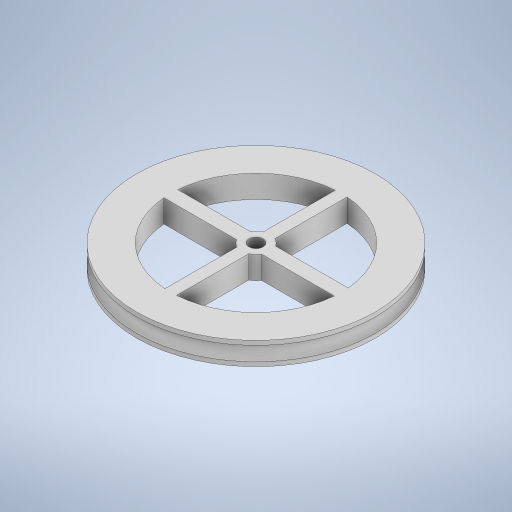
# Autodesk Inventor part: Roue_pami_V3
Saved by Autodesk Inventor 2023 (Build 270158000, 158)
## iProperties
Created: 2024-02-08
Part Number: Roue_pami_V3
Material: Generic
Document SubType Name: Modeling
Designer: eliott
Density: 1 g/cm^3
Appearance: Default
Author: eliott
Autodesk Inventor part; units mm, degrees
ref_plane "YZ Plane" through (0, 0, 0) normal (1, 0, 0) x (0, 1, 0)
ref_plane "XZ Plane" through (0, 0, 0) normal (0, 1, 0) x (-1, 0, 0)
ref_plane "XY Plane" through (0, 0, 0) normal (0, 0, 1) x (1, 0, 0)
sketch "Sketch1" plane through (0, 0, 0) normal (0, 0, 1) x (1, 0, 0)
  line L0 (0, 0) -> (2.5, 0)
  line L1 (2.5, 0) -> (2.5, 8)
  line L2 (2.5, 8) -> (0, 8)
  line L3 (0, 8) -> (0, 0)
  line L4 (2.5, 8) -> (42, 8)
  line L5 (42, 8) -> (42, 0)
  line L6 (42, 0) -> (2.5, 0)
  line L7 (2.5, 0) -> (2.5, 8)
  circle A0 centre (42, 4) radius 2.5
  point P0 (42, 1.5)
  point P1 (42, 6.5)
  dimension "d0" = 8
  dimension "d1" = 2.5
  dimension "d2" = 39.5
  dimension "d3" = 5
  constraints: 16 end point, 4 parallel, 2 horizontal, 2 perpendicular, 1 centre point, 1 midpoint
  measures "d0" distance of L0.end L1.end
  measures "d1" distance of L1.end L2.end
  measures "d2" distance of L1.end L4.end
  measures "d3" diameter of A0
revolve "Revolution1" add sketch "Sketch1" angle 360 about axis through (0, 8, 0) along (0, -1, 0) contours L1 L4 L5 A0 L6
sketch "Sketch2" plane through (0, 8, 0) normal (0, 1, 0) x (1, 0, 0)
  circle A0 centre (0, 0) radius 2.5 projected
  circle A1 centre (0, 0) radius 30
  circle A2 centre (0, 0) radius 5
  line L0 (-4.3623, -2.4434) -> (-29.9003, -2.4434)
  line L1 (-4.3623, 2.4434) -> (-29.9003, 2.4434)
  line L2 (4.3623, 2.4434) -> (29.9003, 2.4434)
  line L3 (4.3623, -2.4434) -> (29.9003, -2.4434)
  line L4 (2.0546, -4.5583) -> (2.0546, -29.9296)
  line L5 (-2.0546, -4.5583) -> (-2.0546, -29.9296)
  line L6 (-2.0546, 4.5583) -> (-2.0546, 60.5512)
  line L7 (2.0546, 4.5583) -> (2.0546, 29.9296)
  point P0 (-2.0546, 29.9296)
  dimension "d5" = 60
  dimension "d6" = 10
  constraints: 16 end point, 6 point on line, 2 coincident, 1 horizontal, 1 perpendicular, 1 vertical, 19 other
extrude "Extrusion1" cut sketch "Sketch2" against normal blind 25 contours L2 A2 L7 A1 | A1 L4 A2 L3 | L6 A2 L1 A1 | A1 L0 A2 L5
body "Solid1"
